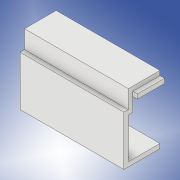
# Autodesk Inventor part: FA003
Saved by Autodesk Inventor 2017 SP1 (Build 210196100, 196)
## iProperties
Created: 2017-06-16
Part Number: FA003
Material: ABS Plastic
Document SubType Name: Modeling
Designer: Zach
Density: 1.06 g/cm^3
Appearance: CR White
Author: Zach
Autodesk Inventor part; units mm, degrees
ref_plane "YZ Plane" through (0, 0, 0) normal (1, 0, 0) x (0, 1, 0)
ref_plane "XZ Plane" through (0, 0, 0) normal (0, 1, 0) x (-1, 0, 0)
ref_plane "XY Plane" through (0, 0, 0) normal (0, 0, 1) x (1, 0, 0)
sketch "Sketch1" plane through (0, 0, 0) normal (0, 0, 1) x (1, 0, 0)
  line L0 (0, 0) -> (115, 0)
  line L1 (115, 0) -> (115, 75)
  line L2 (115, 75) -> (0, 75)
  line L3 (0, 75) -> (0, 0)
  dimension "d0" = 115
  dimension "d1" = 75
  constraints: 8 end point, 2 parallel, 1 horizontal, 1 perpendicular
  measures "d0" distance of L2.end L1.end
  measures "d1" distance of L1.end L0.end
extrude "Extrusion1" add sketch "Sketch1" along normal blind 40
sketch "Sketch2" plane through (0, 0, 40) normal (0, 0, 1) x (1, 0, 0)
  line L0 (115, 75) -> (0, 75) projected
  line L1 (115, 0) -> (115, 75) projected
  line L2 (0, 75) -> (115, 75)
  line L3 (115, 75) -> (115, 55)
  line L4 (115, 55) -> (0, 55)
  line L5 (0, 55) -> (0, 75)
  point P0 (0, 0)
  dimension "d4" = 20
  constraints: 8 end point, 2 parallel, 1 horizontal, 1 perpendicular, 1 point on line
  measures "d4" distance of L2.end L3.end
extrude "Extrusion2" cut sketch "Sketch2" against normal blind 5
sketch "Sketch3" plane through (115, 0, 0) normal (1, 0, 0) x (0, 0, -1)
  line L0 (0, 75) -> (-35, 75) projected
  line L1 (-35, 75) -> (-35, 55) projected
  line L2 (-35, 55) -> (-40, 55) projected
  line L3 (-40, 0) -> (-40, 55) projected
  line L4 (0, 0) -> (-40, 0) projected
  line L5 (0, 70) -> (-30, 70)
  line L6 (-30, 70) -> (-30, 50)
  line L7 (-30, 50) -> (-35, 50)
  line L8 (-35, 50) -> (-35, 5)
  line L9 (-35, 5) -> (0, 5)
  line L10 (0, 5) -> (0, 70)
  line L11 (0, 0) -> (0, 75) projected
  dimension "d7" = 5
  constraints: 12 end point, 1 collinear, 4 other
  measures "d7" distance between parallel lines of L0 L5
extrude "Extrusion3" cut sketch "Sketch3" against normal through all contours L10 L9 L8 L7 L6 L5
sketch "Sketch4" plane through (115, 5, 35) normal (0, 0, -1) x (-1, 0, 0)
  line L0 (0, 45) -> (115, 45) projected
  line L1 (115, 0) -> (0, 0) projected
  line L2 (115, 45) -> (110, 45)
  line L3 (110, 45) -> (110, 0)
  line L4 (110, 0) -> (115, 0)
  line L5 (115, 0) -> (115, 45)
  point P0 (115, -5)
  dimension "d10" = 5
  constraints: 8 end point, 2 parallel, 1 horizontal, 1 perpendicular, 1 point on line
  measures "d10" distance of L4.end L3.end
extrude "Extrusion4" add sketch "Sketch4" along normal blind 5
sketch "Sketch5" plane through (115, 50, 30) normal (0, 0, -1) x (-1, 0, 0)
  line L0 (115, 20) -> (115, -45) projected
  line L1 (115, -45) -> (110, -45)
  line L2 (110, -45) -> (110, 0)
  line L3 (110, 0) -> (115, 0)
  line L4 (115, 0) -> (115, -45)
  point P0 (115, -50)
  dimension "d13" = 5
  dimension "d14" = 45
  constraints: 8 end point, 2 parallel, 1 horizontal, 1 perpendicular
  measures "d13" distance of L2.end L3.end
  measures "d14" distance of L1.end L2.end
extrude "Extrusion5" add sketch "Sketch5" along normal blind 30
sketch "Sketch6" plane through (0, 0, 0) normal (0, 0, -1) x (-1, 0, 0)
  line L0 (-5, 5) -> (-5, 50) projected
  line L1 (-5, 5) -> (-50, 5)
  line L2 (-50, 5) -> (-50, 50)
  line L3 (-50, 50) -> (-5, 50)
  line L4 (-5, 50) -> (-5, 5)
  point P0 (0, 0)
  dimension "d17" = 45
  dimension "d18" = 45
  constraints: 8 end point, 2 parallel, 1 horizontal, 1 perpendicular
  measures "d17" distance of L2.end L3.end
  measures "d18" distance of L1.end L2.end
extrude "Extrusion6" add sketch "Sketch6" against normal blind 5
sketch "Sketch7" plane through (0, 0, 0) normal (0, 0, -1) x (-1, 0, 0)
  line L0 (0, 50) -> (-50, 50) construction
  line L1 (-5, 5) -> (-5, 50) construction
  line L2 (-50, 50) -> (-5, 50) construction
  line L3 (-5, 50) -> (-5, 5) construction
  line L4 (-5, 5) -> (-50, 5) construction
  line L5 (-50, 5) -> (-50, 50) construction
  line L6 (-43, 12) -> (-12, 12) construction
  line L7 (-12, 12) -> (-12, 43) construction
  line L8 (-12, 43) -> (-43, 43) construction
  line L9 (-43, 43) -> (-43, 12) construction
  line L10 (-43, 12) -> (-12, 43) construction
  line L11 (-12, 12) -> (-43, 43) construction
  circle A0 centre (-43, 43) radius 1.5
  circle A1 centre (-12, 43) radius 1.5
  circle A2 centre (-43, 12) radius 1.5
  circle A3 centre (-12, 12) radius 1.5
  circle A4 centre (-27.5, 27.5) radius 3
  point P0 (0, 0)
  point P1 (-50, 27.5)
  point P2 (-27.5, 50)
  dimension "d21" = 45
  dimension "d22" = 45
  dimension "d23" = 31
  dimension "d24" = 31
  dimension "d25" = 3
  dimension "d26" = 3
  dimension "d27" = 3
  dimension "d28" = 3
  dimension "d29" = 6
  constraints: 20 end point, 6 midpoint, 5 centre point, 5 coincident, 4 parallel, 2 horizontal, 2 perpendicular, 1 horizontal alignment, 1 vertical alignment
  measures "d21" distance of L1.start L4.end
  measures "d22" distance of L2.end L1.start
  measures "d23" distance of L8.end L7.end
  measures "d24" distance of L7.end L6.end
  measures "d25" diameter of A0
  measures "d26" diameter of A1
  measures "d27" diameter of A2
  measures "d28" diameter of A3
  measures "d29" diameter of A4
extrude "Extrusion7" cut sketch "Sketch7" against normal blind 5
sketch "Sketch8" plane through (0, 0, 0) normal (0, 0, -1) x (-1, 0, 0)
  circle A0 centre (-27.5, 27.5) radius 3 projected
  circle A1 centre (-27.5, 27.5) radius 12.5
  point P0 (0, 0)
  dimension "d32" = 25
  constraints: 1 centre point, 1 coincident
  measures "d32" diameter of A1
extrude "Extrusion8" cut sketch "Sketch8" against normal blind 2
sketch "Sketch9" plane through (115, 50, 30) normal (0, 0, -1) x (-1, 0, 0)
  line L0 (115, 5) -> (115, -50) projected
  line L1 (115, 0) -> (65, 0)
  line L2 (65, 0) -> (65, 5)
  line L3 (65, 5) -> (115, 5)
  line L4 (115, 5) -> (115, 0)
  dimension "d35" = 50
  dimension "d36" = 5
  constraints: 8 end point, 2 parallel, 1 horizontal, 1 perpendicular
  measures "d35" distance of L2.end L3.end
  measures "d36" distance of L1.end L2.end
extrude "Extrusion9" add sketch "Sketch9" along normal blind 30
sketch "Sketch10" plane through (115, 5, 35) normal (0, 0, -1) x (-1, 0, 0)
  circle A0 centre (87.5, 22.5) radius 3 projected
  circle A1 centre (87.5, 22.5) radius 12.5
  point P0 (115, -5)
  dimension "d39" = 25
  constraints: 1 centre point, 1 coincident
  measures "d39" diameter of A1
extrude "Extrusion10" add sketch "Sketch10" along normal blind 5 contours A0 | A1
sketch "Sketch11" plane through (0, 0, 0) normal (0, 0, -1) x (-1, 0, 0)
  line L0 (-120, 70) -> (5, 70)
  line L1 (5, 70) -> (5, 65)
  line L2 (5, 65) -> (-120, 65)
  line L3 (-120, 65) -> (-120, 70)
  line L4 (-115, 70) -> (-115, 75) projected
  point P0 (0, 0)
  point P1 (0, 70)
  dimension "d42" = 5
  dimension "d43" = 5
  dimension "d44" = 5
  constraints: 8 end point, 2 parallel, 1 horizontal, 1 horizontal alignment, 1 perpendicular
  measures "d42" distance of L0.end L1.end
  measures "d43" distance of L0.end point (0, 70)
  measures "d44" distance from line of L4 L0.start
extrude "Extrusion11" add sketch "Sketch11" against normal blind 30
body "Solid1"
